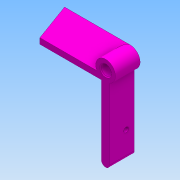
# Autodesk Inventor part: Pancake_Switch Lever
Saved by Autodesk Inventor 2018.1 (Build 221171000, 171)
## iProperties
Created: 2019-03-01
Part Number: Pancake_Switch Lever
Material: ABS Plastic
Document SubType Name: Modeling
Designer: James
Density: 1.06 g/cm^3
Appearance: Magenta
Author: James
Autodesk Inventor part; units mm, degrees
ref_plane "XZ Plane" through (0, 0, 0) normal (0, 1, 0) x (-1, 0, 0)
ref_plane "XY Plane" through (0, 0, 0) normal (0, 0, 1) x (1, 0, 0)
sketch "Sketch1" plane through (0, 0, 0) normal (0, 1, 0) x (-1, 0, 0)
  circle A0 centre (0, 0) radius 6
  line L0 (-2.5, 0) -> (2.5, 0)
  line L1 (2.5, 0) -> (2.5, -51)
  line L2 (2.5, -51) -> (-2.5, -51)
  line L3 (-2.5, -51) -> (-2.5, 0)
  dimension "d0" = 12
  dimension "d1" = 5
  dimension "d3" = 51
  constraints: 8 end point, 2 coincident, 2 parallel, 1 centre point, 1 horizontal, 1 midpoint, 1 perpendicular
  measures "d0" diameter of A0
  measures "d1" distance of L0.start L0.end
  measures "d3" distance of L0.end L1.end
extrude "Extrusion1" add sketch "Sketch1" along normal blind 15
ref_plane "Work Plane1" through (0, 0, 0) normal (1, 0, 0) x (0, 1, 0)
sketch "Sketch2" plane through (0, 0, 0) normal (1, 0, 0) x (0, 1, 0)
  line L0 (15, -5.4544) -> (0, -5.4544) projected
  line L1 (0, -5.4544) -> (0, -5.4544) projected
  line L2 (0, -5.4544) -> (15, -5.4544) projected
  line L3 (15, 2.5359) -> (15, 6)
  line L4 (15, 6) -> (0, -2.6603)
  line L5 (0, 6) -> (0, -5.4544) projected
  line L6 (0, -2.6603) -> (0, -6.1244)
  line L7 (0, -6.1244) -> (15, 2.5359)
  line L8 (0, 6) -> (15, 6) projected
  line L9 (15, -5.4544) -> (15, 6) projected
  point P0 (0, 0)
  point P1 (10.5616, 3.716)
  dimension "d7" = 3
  dimension "d9" = 60
  dimension "d19" = 0
  constraints: 8 end point, 2 point on line, 1 collinear, 1 parallel, 1 vertical, 1 other
  measures "d7" distance between parallel lines of L4 L7
  measures "d9" angle of L3 L7
extrude "Extrusion2" add sketch "Sketch2" against normal blind 40 contours L7 L6 L0 | L0 L5 L4 L3 L7
full round fillet "Fillet1" first side at (-2.5, 10, -20.8596) centre faces at (-0.8333, 5, -51) second side at (2.5, 5, -35.8181)
sketch "Sketch3" plane through (0, 15, 0) normal (0, 1, 0) x (1, 0, 0)
  point P0 (0, 0)
  point P1 (0, 0)
  constraints: 1 coincident
hole "Hole1" at (0, 15, 0) direction (0, -1, 0) diameter 6.2 end through all
chamfer "Chamfer1" distance 0.5 angle 45 1 edges at (0, 0, -3.1)
sketch "Sketch4" plane through (-2.5, 1.1605, -5.4544) normal (-1, 0, 0) x (0, 0, 1)
  line L0 (-43.0456, 13.8395) -> (0, 13.8395) projected
  line L1 (5.4544, -4.1605) -> (5.4544, 16.8395) projected
  point P0 (5.4544, -1.1605)
  point P1 (-29.5456, 8.8395)
  dimension "d23" = 5
  dimension "d24" = 35
  measures "d23" distance from line of L0 point (-29.546, 8.84)
  measures "d24" distance from line of L1 point (-29.546, 8.84)
hole "Hole2" at (-2.5, 10, -35) direction (1, 0, 0) diameter 3 end through all
body "Solid1"
